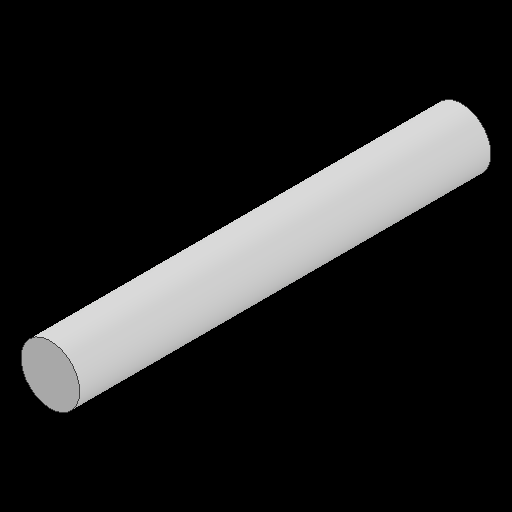
# Autodesk Inventor part: pasador
Saved by Autodesk Inventor 2027 (Build 310192000, 192)
## iProperties
Created: 2026-05-13
Part Number: pasador
Material: Genérico
Document SubType Name: Modeling
Designer: giova
Density: 1 g/cm^3
Appearance: Valor por defecto
Author: giova
Autodesk Inventor part; units mm, degrees
ref_plane "YZ Plane" through (0, 0, 0) normal (1, 0, 0) x (0, 1, 0)
ref_plane "XZ Plane" through (0, 0, 0) normal (0, 1, 0) x (-1, 0, 0)
ref_plane "XY Plane" through (0, 0, 0) normal (0, 0, 1) x (1, 0, 0)
sketch "Boceto1" plane through (0, 0, 0) normal (0, 0, 1) x (1, 0, 0)
  circle A0 centre (0, 0) radius 2.5
  dimension "d2" = 5
  dimension "d2" = 5
  constraints: 1 centre point
  measures "d2" diameter of A0
extrude "Extrusión1" add sketch "Boceto1" along normal blind 35
